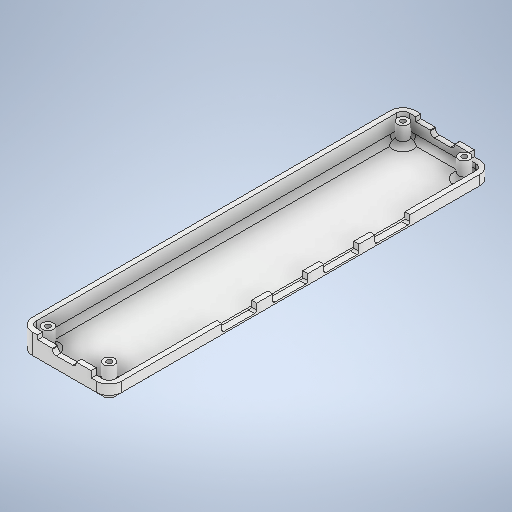
# Autodesk Inventor part: Upper_Housing
Saved by Autodesk Inventor 2025.1 (Build 291241020, 241B)
## iProperties
Created: 2026-01-18
Part Number: Upper_Housing
Material: Resina de poliariletercetona
Document SubType Name: Modeling
Designer: JoaoVitorRamosMitidi
Density: 1.32 g/cm^3
Appearance: Suave - Branco
Author: JoaoVitorRamosMitidi
Autodesk Inventor part; units mm, degrees
ref_plane "YZ Plane" through (0, 0, 0) normal (1, 0, 0) x (0, 1, 0)
ref_plane "XZ Plane" through (0, 0, 0) normal (0, 1, 0) x (-1, 0, 0)
ref_plane "XY Plane" through (0, 0, 0) normal (0, 0, 1) x (1, 0, 0)
sketch "Esboço1" plane through (0, 0, 0) normal (0, 1, 0) x (-1, 0, 0)
  line L0 (-12.5, 75) -> (12.5, 75)
  line L1 (17.5, 70) -> (17.5, -70)
  line L2 (12.5, -75) -> (-12.5, -75)
  line L3 (-17.5, -70) -> (-17.5, 70)
  line L4 (-17.5, 75) -> (17.5, -75) construction
  line L5 (17.5, 75) -> (-17.5, -75) construction
  line L6 (-13, 73) -> (13, 73)
  line L7 (15.5, 70.5) -> (15.5, -70.5)
  line L8 (13, -73) -> (-13, -73)
  line L9 (-15.5, -70.5) -> (-15.5, 70.5)
  line L10 (-15.5, 73) -> (15.5, -73) construction
  line L11 (15.5, 73) -> (-15.5, -73) construction
  circle A0 centre (12, 69.5) radius 1
  circle A1 centre (-12, 69.5) radius 1
  circle A2 centre (-12, -69.5) radius 1
  circle A3 centre (12, -69.5) radius 1
  line L12 (-11.2693, 48.2969) -> (11.2693, -48.2969) construction
  line L13 (11.6146, 48.7168) -> (-11.6146, -48.7168) construction
  line L14 (-13, 72.5) -> (13, 72.5)
  line L15 (15, 70.5) -> (15, -70.5)
  line L16 (13, -72.5) -> (-13, -72.5)
  line L17 (-15, -70.5) -> (-15, 70.5)
  line L18 (-15, 72.5) -> (15, -72.5) construction
  line L19 (15, 72.5) -> (-15, -72.5) construction
  arc A4 (-13, 72.5) -> (-15, 70.5) centre (-13, 70.5) ccw
  arc A5 (15, 70.5) -> (13, 72.5) centre (13, 70.5) ccw
  arc A6 (-15, -70.5) -> (-13, -72.5) centre (-13, -70.5) ccw
  arc A7 (13, -72.5) -> (15, -70.5) centre (13, -70.5) ccw
  arc A8 (-13, 73) -> (-15.5, 70.5) centre (-13, 70.5) ccw
  arc A9 (15.5, 70.5) -> (13, 73) centre (13, 70.5) ccw
  arc A10 (13, -73) -> (15.5, -70.5) centre (13, -70.5) ccw
  arc A11 (-15.5, -70.5) -> (-13, -73) centre (-13, -70.5) ccw
  arc A12 (-12.5, 75) -> (-17.5, 70) centre (-12.5, 70) ccw
  arc A13 (17.5, 70) -> (12.5, 75) centre (12.5, 70) ccw
  arc A14 (-17.5, -70) -> (-12.5, -75) centre (-12.5, -70) ccw
  arc A15 (12.5, -75) -> (17.5, -70) centre (12.5, -70) ccw
  circle A16 centre (-12, 69.5) radius 2.15
  circle A17 centre (12, 69.5) radius 2.15
  circle A18 centre (12, -69.5) radius 2.15
  circle A19 centre (-12, -69.5) radius 2.15
  line L20 (10.5, -75) -> (10.5, -73)
  line L21 (10.5, 73) -> (10.5, 75)
  line L22 (-10.5, -75) -> (-10.5, -73)
  line L23 (-10.5, 73) -> (-10.5, 75)
  point P0 (0, 0)
  dimension "d4" = 146
  dimension "d5" = 31
  dimension "d7" = 30
  dimension "d8" = 145
  dimension "d9" = 3
  dimension "d10" = 3
  dimension "d11" = 3
  dimension "d12" = 3
  dimension "d13" = 2
  dimension "d14" = 2
  dimension "d15" = 2.5
  dimension "d16" = 5
  dimension "d21" = 4.3
  dimension "d24" = 7
  dimension "d25" = 7
  dimension "d28" = 7
  dimension "d29" = 7
  dimension "d32" = 2.5
  dimension "d33" = 2.5
  constraints: 48 end point, 33 point on line, 24 point on circle, 24 tangent, 20 centre point, 15 equal radius, 8 midpoint, 7 perpendicular, 6 parallel, 4 coincident, 3 horizontal, 2 horizontal alignment, 2 vertical alignment
  measures "d4" distance of L11.start L10.end
  measures "d5" distance of L10.start L11.start
  measures "d7" distance of L18.start L19.start
  measures "d8" distance of L19.start L18.end
  measures "d9" distance from line of L17 A1.centre
  measures "d10" distance from line of L14 A1.centre
  measures "d11" distance from line of L16 A3.centre
  measures "d12" distance from line of L15 A3.centre
  measures "d13" diameter of A3
  measures "d14" radius of A4
  measures "d15" radius of A8
  measures "d16" radius of A12
  measures "d21" diameter of A19
  measures "d24" distance between parallel lines of L1 L20
  measures "d25" distance between parallel lines of L1 L21
  measures "d28" distance between parallel lines of L3 L23
  measures "d29" distance between parallel lines of L3 L22
  measures "d32" distance between parallel lines of L1 L15
  measures "d33" distance between parallel lines of L14 L0
extrude "Extrusão1" add sketch "Esboço1" along normal blind 3 contours L6 A9 L7 A10 L8 A11 L9 A8 | L14 A5 L15 A7 L16 A6 L17 A4 | A16 | A17 | A18 | A19
extrude "Extrusão2" add sketch "Esboço1" along normal blind 10.463 contours A16 | A17 | A18 | A19
extrude "Extrusão3" add sketch "Esboço1" along normal blind 3 contours L0 L23 L6 A8 L9 A11 L8 L22 L2 A14 L3 A12 | L0 L21 L6 L23 | L0 A13 L1 A15 L2 L20 L8 A10 L7 A9 L6 L21 | L22 L8 L20 L2
extrude "Extrusão5" add sketch "Esboço1" along normal blind 6.86 contours L0 L23 L6 A8 L9 A11 L8 L22 L2 A14 L3 A12
sketch "Esboço2" plane through (17.5, 0, 70) normal (1, 0, 0) x (0, 0, -1)
  line L0 (0, 6.86) -> (140, 6.86) projected
  line L1 (112.78, 6.86) -> (112.78, 4.5)
  line L2 (111.98, 3.7) -> (99.88, 3.7)
  line L3 (99.08, 4.5) -> (99.08, 6.86)
  line L4 (92.78, 6.86) -> (92.78, 4.5)
  line L5 (91.98, 3.7) -> (79.88, 3.7)
  line L6 (79.08, 4.5) -> (79.08, 6.86)
  line L7 (72.78, 6.86) -> (72.78, 4.5)
  line L8 (71.98, 3.7) -> (59.88, 3.7)
  line L9 (59.08, 4.5) -> (59.08, 6.86)
  line L10 (52.78, 6.86) -> (52.78, 4.5)
  line L11 (51.98, 3.7) -> (39.88, 3.7)
  line L12 (39.08, 4.5) -> (39.08, 6.86)
  line L13 (0, 0) -> (140, 0) projected
  line L14 (145, 0) -> (145, 6.86) projected
  line L15 (-5, 0) -> (-5, 6.86) projected
  arc A0 (111.98, 3.7) -> (112.78, 4.5) centre (111.98, 4.5) ccw
  arc A1 (99.08, 4.5) -> (99.88, 3.7) centre (99.88, 4.5) ccw
  arc A2 (91.98, 3.7) -> (92.78, 4.5) centre (91.98, 4.5) ccw
  arc A3 (79.08, 4.5) -> (79.88, 3.7) centre (79.88, 4.5) ccw
  arc A4 (71.98, 3.7) -> (72.78, 4.5) centre (71.98, 4.5) ccw
  arc A5 (59.08, 4.5) -> (59.88, 3.7) centre (59.88, 4.5) ccw
  arc A6 (51.98, 3.7) -> (52.78, 4.5) centre (51.98, 4.5) ccw
  arc A7 (39.08, 4.5) -> (39.88, 3.7) centre (39.88, 4.5) ccw
  point P0 (70, 0)
  point P1 (99.08, 3.7)
  point P2 (92.78, 3.7)
  point P3 (79.08, 3.7)
  point P4 (72.78, 3.7)
  point P5 (59.08, 3.7)
  point P6 (52.78, 3.7)
  point P7 (92.78, 5.68)
  point P8 (52.78, 5.68)
  point P9 (59.08, 5.68)
  dimension "d34" = 3.7
  dimension "d35" = 13.7
  dimension "d36" = 6.3
  dimension "d37" = 6.3
  dimension "d38" = 6.3
  dimension "d39" = 32.22
  dimension "d40" = 44.08
  dimension "d41" = 0.8
  constraints: 24 end point, 16 point on circle, 16 tangent, 12 point on line, 8 centre point, 7 equal radius, 7 vertical, 5 perpendicular, 3 collinear, 3 horizontal alignment, 3 midpoint, 9 other
  measures "d34" distance between parallel lines of L13 L2
  measures "d35" distance between parallel lines of L3 L1
  measures "d36" distance from line of point (92.78, 5.68) L3
  measures "d37" distance between parallel lines of L7 L6
  measures "d38" distance of point (52.78, 5.68) point (59.08, 5.68)
  measures "d39" distance between parallel lines of L14 L1
  measures "d40" distance between parallel lines of L15 L12
  measures "d41" radius of A0
extrude "Extrusão6" cut sketch "Esboço2" against normal up to surface (2 mm away)
extrude "Extrusão7" add sketch "Esboço1" along normal blind 9.35 contours L0 L21 L6 L23
sketch "Esboço3" plane through (-12.5, 0, 75) normal (0, 0, 1) x (1, 0, 0)
  line L0 (2, 9.35) -> (23, 9.35) projected
  line L1 (17.17, 9.35) -> (17.17, 9.05)
  line L2 (15.69, 7.57) -> (9.31, 7.57)
  line L3 (7.83, 9.05) -> (7.83, 9.35)
  line L4 (0, 0) -> (25, 0) projected
  line L5 (30, 0) -> (30, 6.86) projected
  line L6 (-5, 0) -> (-5, 3) projected
  arc A0 (15.69, 7.57) -> (17.17, 9.05) centre (15.69, 9.05) ccw
  arc A1 (7.83, 9.05) -> (9.31, 7.57) centre (9.31, 9.05) ccw
  point P0 (12.5, 0)
  point P1 (17.17, 7.57)
  point P2 (7.83, 7.57)
  point P3 (7.83, 9.2)
  dimension "d46" = 9.34
  dimension "d47" = 7.57
  dimension "d48" = 12.83
  dimension "d49" = 12.83
  dimension "d50" = 1.48
  constraints: 6 end point, 6 point on line, 4 point on circle, 4 tangent, 3 perpendicular, 2 centre point, 1 equal radius, 1 midpoint
  measures "d46" distance of point (17.17, 7.57) point (7.83, 7.57)
  measures "d47" distance between parallel lines of L4 L2
  measures "d48" distance between parallel lines of L5 L1
  measures "d49" distance from line of L6 point (7.83, 9.2)
  measures "d50" radius of A0
extrude "Extrusão8" cut sketch "Esboço3" against normal up to surface (2 mm away)
extrude "Extrusão9" add sketch "Esboço1" along normal blind 9.275 contours L22 L8 L20 L2
sketch "Esboço4" plane through (12.5, 0, -75) normal (0, 0, -1) x (-1, 0, 0)
  line L0 (23, 9.275) -> (2, 9.275) projected
  line L1 (17.27, 9.275) -> (17.27, 8.975)
  line L2 (15.69, 7.395) -> (9.31, 7.395)
  line L3 (7.73, 8.975) -> (7.73, 9.275)
  line L4 (0, 0) -> (25, 0) projected
  line L5 (30, 0) -> (30, 3) projected
  line L6 (-5, 0) -> (-5, 6.86) projected
  arc A0 (15.69, 7.395) -> (17.27, 8.975) centre (15.69, 8.975) ccw
  arc A1 (7.73, 8.975) -> (9.31, 7.395) centre (9.31, 8.975) ccw
  point P0 (12.5, 0)
  point P1 (17.27, 7.395)
  point P2 (7.73, 7.395)
  point P3 (12.5, 7.395)
  dimension "d55" = 9.54
  dimension "d56" = 7.395
  dimension "d57" = 12.73
  dimension "d58" = 12.73
  dimension "d59" = 1.58
  constraints: 6 end point, 6 point on line, 4 point on circle, 4 tangent, 2 centre point, 2 perpendicular, 1 equal radius, 1 midpoint, 1 vertical
  measures "d55" distance of point (17.27, 7.395) point (7.73, 7.395)
  measures "d56" distance from line of L4 point (12.5, 7.395)
  measures "d57" distance between parallel lines of L5 L1
  measures "d58" distance between parallel lines of L6 L3
  measures "d59" radius of A0
extrude "Extrusão10" cut sketch "Esboço4" against normal up to surface (2 mm away)
extrude "Extrusão11" add sketch "Esboço1" along normal blind 10.963 contours L0 A13 L1 A15 L2 L20 L8 A10 L7 A9 L6 L21
extrude "Extrusão12" add sketch "Esboço1" along normal blind 5 contours A0 | A1 | A2 | A3
chamfer "Chanfro1" distance 3 angle 45 8 edges at (17.5, 0, 0) (16.0355, 0, -73.5355) (0, 0, -75) (-16.0355, 0, -73.5355) (-17.5, 0, 0) (-16.0355, 0, 73.5355) (0, 0, 75) (16.0355, 0, 73.5355)
thread "Rosca1" size "M2x0.4" class "6H" standard "ANSI Metric M Profile" full length
thread "Rosca2" size "M2x0.4" class "6H" standard "ANSI Metric M Profile" full length
thread "Rosca3" size "M2x0.4" class "6H" standard "ANSI Metric M Profile" full length
thread "Rosca4" size "M2x0.4" class "6H" standard "ANSI Metric M Profile" full length
fillet "Arredondamento1" radius 2 12 edges at (-14.7678, 3, -72.2678) (-15.5, 3, 0) (-14.7678, 3, 72.2678) (0, 3, 73) (14.7678, 3, 72.2678) (15.5, 3, 0) (14.7678, 3, -72.2678) (0, 3, -73) (14.15, 3, -69.5) (-9.85, 3, -69.5) (-9.85, 3, 69.5) (14.15, 3, 69.5)
